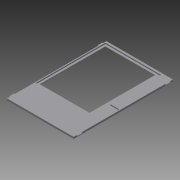
# Autodesk Inventor part: TopTouch
Saved by Autodesk Inventor 2014 SP1 (Build 180222100, 222)
## iProperties
Created: 2014-03-24
Part Number: TopTouch
Material: Generic
Document SubType Name: Modeling
Designer: patrigg
Density: 1 g/cm^3
Appearance: Default
Author: patrigg
Autodesk Inventor part; units mm, degrees
ref_plane "YZ Plane" through (0, 0, 0) normal (1, 0, 0) x (0, 1, 0)
ref_plane "XZ Plane" through (0, 0, 0) normal (0, 1, 0) x (-1, 0, 0)
ref_plane "XY Plane" through (0, 0, 0) normal (0, 0, 1) x (1, 0, 0)
sketch "Sketch1" plane through (0, 0, 0) normal (0, 1, 0) x (-1, 0, 0)
  line L0 (-33.5, -50) -> (33.5, -50)
  line L1 (33.5, -50) -> (33.5, 50)
  line L2 (33.5, 50) -> (-33.5, 50)
  line L3 (-33.5, 50) -> (-33.5, -50)
  line L4 (-33.5, -50) -> (33.5, 50) construction
  line L5 (33.5, -50) -> (-33.5, 50) construction
  point P0 (0, 0)
  dimension "d0" = 67
  dimension "d1" = 100
  constraints: 12 end point, 2 midpoint, 2 parallel, 1 horizontal, 1 perpendicular
  measures "d0" distance of L2.end L1.end
  measures "d1" distance of L1.end L0.end
extrude "Extrusion1" add sketch "Sketch1" along normal blind 1.8
sketch "Sketch2" plane through (0, 1.8, 0) normal (0, 1, 0) x (1, 0, 0)
  line L0 (33.5, 50) -> (-33.5, 50) projected
  line L1 (-32.5, -22) -> (23.5, -22)
  line L2 (23.5, -22) -> (23.5, 48)
  line L3 (23.5, 48) -> (-32.5, 48)
  line L4 (-32.5, 48) -> (-32.5, -22)
  line L5 (-32.5, -22) -> (23.5, 48) construction
  line L6 (23.5, -22) -> (-32.5, 48) construction
  line L7 (-33.5, 50) -> (-33.5, -50) projected
  point P0 (0, 0)
  point P1 (-4.5, 13)
  point P2 (-4.5, 13)
  dimension "d5" = 56
  dimension "d6" = 70
  dimension "d7" = 2
  dimension "d22" = 1
  constraints: 12 end point, 3 midpoint, 2 parallel, 1 horizontal, 1 perpendicular
  measures "d5" distance of L3.end L2.end
  measures "d6" distance of L2.end L1.end
  measures "d7" distance between parallel lines of L0 L3
  measures "d22" distance between parallel lines of L7 L4
extrude "Extrusion2" cut sketch "Sketch2" against normal blind 1.1
sketch "Sketch3" plane through (0, 0.7, 0) normal (0, 1, 0) x (1, 0, 0)
  line L0 (23.5, -22) -> (-32.5, -22) projected
  line L1 (23.5, 48) -> (23.5, -22) projected
  line L2 (-32.5, 48) -> (23.5, 48) projected
  line L3 (-32.5, -22) -> (-32.5, 48) projected
  line L4 (-30.5, 46) -> (19.5, 46)
  line L5 (19.5, 46) -> (19.5, -20)
  line L6 (19.5, -20) -> (-30.5, -20)
  line L7 (-30.5, -20) -> (-30.5, 46)
  point P0 (0, 0)
  dimension "d10" = 2
  dimension "d11" = 2
  dimension "d12" = 4
  dimension "d13" = 2
  constraints: 8 end point, 2 parallel, 1 horizontal, 1 perpendicular
  measures "d10" distance between parallel lines of L2 L4
  measures "d11" distance between parallel lines of L3 L7
  measures "d12" distance between parallel lines of L1 L5
  measures "d13" distance between parallel lines of L0 L6
extrude "Extrusion3" cut sketch "Sketch3" against normal blind 1 contours L4 L5 L6 L7
sketch "Sketch4" plane through (0, 1.8, 0) normal (0, 1, 0) x (1, 0, 0)
  line L0 (23.5, 48) -> (23.5, -22) projected
  line L1 (23.5, -22) -> (-32.5, -22) projected
  line L2 (33.5, -50) -> (33.5, 50) projected
  line L3 (23.5, -3) -> (32.5, -3)
  line L4 (32.5, -3) -> (32.5, -18)
  line L5 (32.5, -18) -> (23.5, -18)
  line L6 (23.5, -18) -> (23.5, -3)
  point P0 (0, 0)
  dimension "d16" = 4
  dimension "d18" = 1
  dimension "d21" = 15
  constraints: 8 end point, 2 parallel, 1 horizontal, 1 perpendicular, 1 point on line
  measures "d16" distance between parallel lines of L1 L5
  measures "d18" distance between parallel lines of L2 L4
  measures "d21" distance between parallel lines of L3 L5
extrude "Extrusion4" cut sketch "Sketch4" against normal up to surface (1.1 mm away)
sketch "Sketch6" plane through (33.5, 0, 50) normal (1, 0, 0) x (0, 0, -1)
  line L0 (100, 0) -> (100, 1.8) projected
  line L1 (0, 1.8) -> (100, 1.8) projected
  line L2 (0, 0) -> (0, 1.8) projected
  line L3 (3, 1.8) -> (8, 1.8)
  line L4 (8, 1.8) -> (8, 0.8)
  line L5 (8, 0.8) -> (3, 0.8)
  line L6 (3, 0.8) -> (3, 1.8)
  line L7 (92, 1.8) -> (97, 1.8)
  line L8 (97, 1.8) -> (97, 0.8)
  line L9 (97, 0.8) -> (92, 0.8)
  line L10 (92, 0.8) -> (92, 1.8)
  point P0 (50, 0)
  dimension "d23" = 5
  dimension "d24" = 1
  dimension "d25" = 3
  dimension "d26" = 5
  dimension "d27" = 1
  dimension "d28" = 3
  constraints: 16 end point, 4 parallel, 2 horizontal, 2 perpendicular, 2 point on line
  measures "d23" distance of L4.end L5.end
  measures "d24" distance of L3.end L4.end
  measures "d25" distance between parallel lines of L6 L2
  measures "d26" distance of L8.end L9.end
  measures "d27" distance of L7.end L8.end
  measures "d28" distance between parallel lines of L0 L8
extrude "Extrusion5" add sketch "Sketch6" along normal blind 1 draft -10
sketch "Sketch7" plane through (-33.5, 0, -50) normal (-1, 0, 0) x (0, 0, 1)
  line L0 (92, 0.8) -> (97, 0.8) projected
  line L1 (97, 0.8) -> (97, 1.8) projected
  line L2 (97, 1.8) -> (92, 1.8) projected
  line L3 (92, 1.8) -> (92, 0.8) projected
  line L4 (3, 1.8) -> (3, 0.8) projected
  line L5 (8, 1.8) -> (3, 1.8) projected
  line L6 (3, 0.8) -> (8, 0.8) projected
  line L7 (8, 0.8) -> (8, 1.8) projected
  point P0 (50, 0)
extrude "Extrusion6" add sketch "Sketch7" along normal blind 1 draft -10
body "Solid1"
